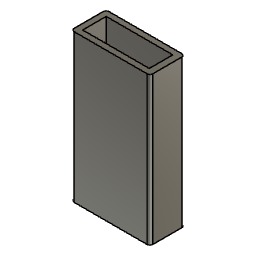
boitier_batterie (Autodesk Fusion 360 design; units mm, degrees)
Autodesk Fusion 360 part; units mm, degrees
sketch "Esquisse1" plane through (0, 0, 0) normal (0, 0, 1) x (1, 0, 0)
  line L0 (0, 0) -> (69.8, 0)
  line L1 (69.8, 0) -> (69.8, 24.65)
  line L2 (69.8, 24.65) -> (0, 24.65)
  line L3 (0, 24.65) -> (0, 0)
  line L4 (-3, -6) -> (73.5, -6)
  line L5 (76.5, -3) -> (76.5, 27.5)
  line L6 (73.5, 30.5) -> (-3, 30.5)
  line L7 (-6, 27.5) -> (-6, -3)
  arc A0 (-3, 30.5) -> (-6, 27.5) centre (-3, 27.5) ccw
  arc A1 (-6, -3) -> (-3, -6) centre (-3, -3) ccw
  arc A2 (76.5, 27.5) -> (73.5, 30.5) centre (73.5, 27.5) ccw
  arc A3 (73.5, -6) -> (76.5, -3) centre (73.5, -3) ccw
  circle A4 centre (12.4, 12.325) radius 3
  circle A5 centre (57.4, 12.325) radius 3
  line L8 (12.4, 15.325) -> (57.4, 15.325)
  line L9 (57.4, 15.325) -> (57.4, 9.325)
  line L10 (57.4, 9.325) -> (12.4, 9.325)
  line L11 (12.4, 9.325) -> (12.4, 15.325)
  dimension "d1" = 69.8
  dimension "d2" = 24.65
  dimension "d33" = 3
  dimension "d34" = 3
  dimension "d35" = 3
  dimension "d36" = 3
  dimension "d39" = 6
  dimension "d42" = 45
  dimension "d43" = 0
  dimension "d52" = 12.4
  dimension "d53" = 12.4
  dimension "d54" = 6
  dimension "d55" = 9.325
  constraint horizontal L0
  constraint vertical L1
  constraint horizontal L2
  constraint vertical L3
  constraint coincident L0.start L3.end
  constraint parallel L0 L4
  constraint parallel L1 L5
  constraint parallel L2 L6
  constraint parallel L3 L7
  constraint tangent L6 A0
  constraint tangent L7 A0
  constraint tangent L4 A1
  constraint tangent L7 A1
  constraint tangent L5 A2
  constraint tangent L6 A2
  constraint tangent L4 A3
  constraint tangent L5 A3
  constraint horizontal L8
  constraint vertical L9
  constraint horizontal L10
  constraint vertical L11
  constraint coincident A5 L9.end
  constraint coincident A4 L8.start
  measures "d1" distance of L0.start L0.end
  measures "d2" distance of L0.start L2.end
  measures "d33" radius of A0
  measures "d34" radius of A1
  measures "d35" radius of A2
  measures "d36" radius of A3
  measures "d39" diameter of A4
  measures "d52" distance of L1 A5.centre
  measures "d53" distance of L3 A4.centre
  measures "d54" distance of L8 L10
  measures "d55" distance of L0 L10
extrude "Extrusion1" add sketch "Esquisse1" along normal blind 6 contours L0 L1 L2 L3 | A4 L11 | A4 A5 L8 L10 | A4 L11 | A5 L9 | A5 L9
extrude "Extrusion2" add sketch "Esquisse1" along normal blind 154.9 contours L4 L5 L6 L7 A0 A1 A2 A3
sketch "Esquisse2" plane through (0, 30.5, 0) normal (0, 1, 0) x (-1, 0, 0)
  line L0 (-73.5, 0) -> (3, 0)
  line L1 (3, 154.9) -> (-73.5, 154.9)
  line L2 (-5, 110) -> (-15, 110)
  line L3 (-15, 110) -> (-15, 100)
  line L4 (-15, 100) -> (-5, 100)
  line L5 (-5, 100) -> (-5, 110)
  line L6 (-15, 100) -> (-10, 100)
  line L7 (-10, 100) -> (-10, 105)
  line L8 (-10, 105) -> (-15, 105)
  line L9 (-15, 105) -> (-15, 100)
  line L10 (-55, 110) -> (-65, 110)
  line L11 (-65, 110) -> (-65, 100)
  line L12 (-65, 100) -> (-55, 100)
  line L13 (-55, 100) -> (-55, 110)
  line L14 (-55, 100) -> (-60, 100)
  line L15 (-60, 100) -> (-60, 105)
  line L16 (-60, 105) -> (-55, 105)
  line L17 (-55, 105) -> (-55, 100)
  line L18 (-4.9962, 35) -> (-14.9962, 35)
  line L19 (-14.9962, 35) -> (-14.9962, 25)
  line L20 (-14.9962, 25) -> (-4.9962, 25)
  line L21 (-4.9962, 25) -> (-4.9962, 35)
  line L22 (-14.9962, 35) -> (-9.9962, 35)
  line L23 (-9.9962, 35) -> (-9.9962, 30)
  line L24 (-9.9962, 30) -> (-14.9962, 30)
  line L25 (-14.9962, 30) -> (-14.9962, 35)
  line L26 (-55, 35) -> (-65, 35)
  line L27 (-65, 35) -> (-65, 25)
  line L28 (-65, 25) -> (-55, 25)
  line L29 (-55, 25) -> (-55, 35)
  line L30 (-55, 35) -> (-60, 35)
  line L31 (-60, 35) -> (-60, 30)
  line L32 (-60, 30) -> (-55, 30)
  line L33 (-55, 30) -> (-55, 35)
  line L34 (3, 0) -> (3, 154.9)
  line L35 (-73.5, 154.9) -> (-73.5, 0)
  dimension "d8" = 10
  dimension "d9" = 10
  dimension "d10" = 5
  dimension "d11" = 5
  dimension "d12" = 10
  dimension "d13" = 10
  dimension "d14" = 5
  dimension "d15" = 5
  dimension "d16" = 40
  dimension "d20" = 10
  dimension "d21" = 10
  dimension "d22" = 5
  dimension "d23" = 5
  dimension "d25" = 85
  dimension "d26" = 10
  dimension "d27" = 10
  dimension "d28" = 5
  dimension "d29" = 5
  dimension "d32" = 35
  constraint horizontal L2
  constraint vertical L3
  constraint horizontal L4
  constraint vertical L5
  constraint horizontal L6
  constraint vertical L7
  constraint horizontal L8
  constraint vertical L9
  constraint horizontal L10
  constraint vertical L11
  constraint horizontal L12
  constraint vertical L13
  constraint horizontal L14
  constraint vertical L15
  constraint horizontal L16
  constraint vertical L17
  constraint collinear L2 L10
  constraint horizontal L18
  constraint vertical L19
  constraint horizontal L20
  constraint vertical L21
  constraint horizontal L22
  constraint vertical L23
  constraint horizontal L24
  constraint vertical L25
  constraint horizontal L26
  constraint vertical L27
  constraint horizontal L28
  constraint vertical L29
  constraint horizontal L30
  constraint vertical L31
  constraint horizontal L32
  constraint vertical L33
  constraint collinear L18 L26
  constraint collinear L11 L27
  measures "d8" distance of L2.start L2.end
  measures "d9" distance of L2.start L4.end
  measures "d10" distance of L3.end L6.end
  measures "d11" distance of L3.end L8.end
  measures "d12" distance of L10.start L10.end
  measures "d13" distance of L10.start L12.end
  measures "d14" distance of L12.end L14.end
  measures "d15" distance of L12.end L16.end
  measures "d16" distance of L3 L13
  measures "d20" distance of L18.start L18.end
  measures "d21" distance of L18.start L20.end
  measures "d22" distance of L18.end L22.end
  measures "d23" distance of L18.end L24.end
  measures "d25" distance of L2 L20
  measures "d26" distance of L26.start L26.end
  measures "d27" distance of L26.start L28.end
  measures "d28" distance of L26.start L30.end
  measures "d29" distance of L26.start L32.end
  measures "d32" distance of L0 L22
extrude "Extrusion3" add sketch "Esquisse2" against normal blind 5 contours L2 L3 L4 L5 L7 L8 | L10 L11 L12 L13 L15 L16 | L18 L19 L20 L21 L23 L24 | L26 L27 L28 L29 L31 L32
extrude "Extrusion4" cut sketch "Esquisse2" against normal blind 3 contours L2 L3 L4 L5 L7 L8 | L10 L11 L12 L13 L15 L16 | L18 L19 L20 L21 L23 L24 | L26 L27 L28 L29 L31 L32
extrude "Extrusion5" cut sketch "Esquisse1" along normal blind 9 contours A4 L11 | A4 A5 L8 L10 | A4 L11 | A5 L9 | A5 L9
equation "d6 = 6 mm + 148.9 mm"
equation "d9 = d8"
equation "d10 = d11"
equation "d12 = d8"
equation "d13 = d8"
equation "d14 = d11"
equation "d15 = d11"
equation "d20 = d8"
equation "d21 = d8"
equation "d22 = d11"
equation "d23 = d11"
equation "d26 = d8"
equation "d27 = d8"
equation "d28 = d11"
equation "d29 = d11"
equation "d51 = 45.00 mm"
equation "d52 = ( d1 - d51 ) / 2"
equation "d55 = ( d2 - d54 ) / 2"
